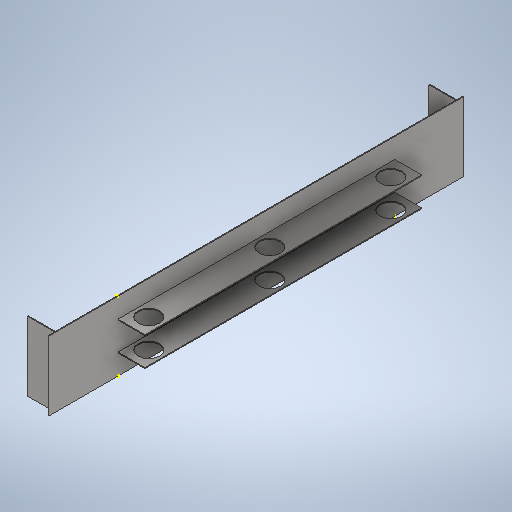
# Autodesk Inventor part: claw platform
Saved by Autodesk Inventor 2025.2 (Build 292293000, 293)
## iProperties
Created: 2025-02-04
Part Number: claw platform
Material: Steel, Galvanized
Document SubType Name: Sheet Metal
Designer: nandu
Density: 7.85 g/cm^3
Sheet Metal Rule: Default_mm
Appearance: Galvanized
Author: nandu
Autodesk Inventor part; units mm, degrees
ref_plane "YZ Plane" through (0, 0, 0) normal (1, 0, 0) x (0, 1, 0)
ref_plane "XZ Plane" through (0, 0, 0) normal (0, 1, 0) x (-1, 0, 0)
ref_plane "XY Plane" through (0, 0, 0) normal (0, 0, 1) x (1, 0, 0)
sketch "Sketch1" plane through (0, 0, 0) normal (1, 0, 0) x (0, 1, 0)
  line L0 (0, 0) -> (50, 0)
  line L1 (50, 0) -> (50, -200)
  line L2 (50, -200) -> (0, -200)
  line L3 (0, -200) -> (0, 0)
  dimension "d0" = 50
  dimension "d1" = 200
  constraints: 8 end point, 2 parallel, 1 horizontal, 1 perpendicular
  measures "d0" distance of L1.end L2.end
  measures "d1" distance of L0.end L1.end
extrude "Extrusion1" add sketch "Sketch1" along normal blind 0.602
sketch "Sketch2" plane through (0.602, 0, 0) normal (1, 0, 0) x (0, 0, -1)
  line L0 (200, 50) -> (0, 50) projected
  line L1 (0, 50) -> (100, 50)
  line L2 (100, 50) -> (100, 35)
  line L3 (0, 0) -> (100, 0)
  line L4 (100, 0) -> (100, 15)
  line L5 (100, 35) -> (200, 35)
  line L6 (200, 0) -> (200, 50) projected
  line L7 (200, 35) -> (200, 35.602)
  line L8 (200, 35.602) -> (0, 35.602)
  line L9 (0, 50) -> (0, 0) projected
  line L10 (0, 35.602) -> (0, 35)
  line L11 (0, 35) -> (100, 35)
  line L12 (100, 15) -> (200, 15)
  line L13 (200, 15) -> (200, 14.398)
  line L14 (200, 14.398) -> (0, 14.398)
  line L15 (0, 14.398) -> (0, 15)
  line L16 (0, 15) -> (100, 15)
  dimension "d4" = 100
  dimension "d5" = 15
  dimension "d6" = 100
  dimension "d7" = 15
  dimension "d9" = 200
  dimension "d13" = 200
  constraints: 28 end point, 6 point on line, 5 perpendicular, 2 horizontal, 1 midpoint, 1 parallel
  measures "d4" distance of L0.end L1.end
  measures "d5" distance of L1.end L2.end
  measures "d6" distance of L3.start L3.end
  measures "d7" distance of L3.end L4.end
  measures "d9" distance of L7.end L8.end
  measures "d13" distance of L13.end L14.end
extrude "Extrusion2" add sketch "Sketch2" along normal blind 19.398 contours L6 L5 L2 L8 | L2 L11 L9 L8 | L6 L14 L4 L12 | L4 L14 L9 L16
sketch "Sketch4" plane through (0.602, 35.602, 0) normal (0, 1, 0) x (1, 0, 0)
  line L0 (-0.602, 0) -> (0, 0) projected
  line L1 (0, 0) -> (0, 12.5)
  line L2 (0, 5) -> (0, 0) projected
  line L3 (0, 12.5) -> (9.699, 12.5)
  line L4 (9.699, 12.5) -> (9.699, 100)
  line L5 (9.699, 100) -> (9.699, 187.5)
  circle A0 centre (9.699, 12.5) radius 7.75
  circle A1 centre (9.699, 100) radius 7.75
  circle A2 centre (9.699, 187.5) radius 7.75
  dimension "d33" = 12.5
  dimension "d34" = 9.699
  dimension "d39" = 15.5
  dimension "d40" = 15.5
  dimension "d41" = 15.5
  dimension "d49" = 87.5
  dimension "d50" = 87.5
  constraints: 8 end point, 3 centre point, 3 coincident, 2 collinear, 2 perpendicular
  measures "d33" distance of L0.end L1.end
  measures "d34" distance of L1.end L3.end
  measures "d39" diameter of A0
  measures "d40" diameter of A1
  measures "d41" diameter of A2
  measures "d49" distance of L5.end L4.end
  measures "d50" distance of L3.end L4.end
extrude "Extrusion4" cut sketch "Sketch4" against normal through all
sketch "Sketch6" plane through (0.602, 15, -200) normal (0, 0, -1) x (-1, 0, 0)
  point P0 (0.602, -15)
sketch "Sketch7" plane through (0, 0, -200) normal (0, 0, -1) x (-1, 0, 0)
  point P0 (0, 0)
sketch "Sketch8" plane through (0, 0, -200) normal (0, 0, -1) x (-1, 0, 0)
  line L0 (-0.602, 50) -> (-0.602, 35.602) projected
  line L1 (-0.602, 50) -> (-0.602, 0)
  line L2 (-0.602, 0) -> (0, 0)
  line L3 (0, 0) -> (0, 50)
  line L4 (0, 50) -> (-0.602, 50)
  constraints: 8 end point, 3 perpendicular, 1 vertical
extrude "Extrusion6" add sketch "Sketch8" along normal blind 50
sketch "Sketch9" plane through (0, 0, 0) normal (0, 0, 1) x (1, 0, 0)
  line L0 (0, 0) -> (0, 50) projected
  line L1 (0, 0) -> (0, 50)
  line L2 (0, 50) -> (0.602, 50)
  line L3 (0.602, 50) -> (0.602, 0)
  line L4 (0.602, 0) -> (0, 0)
  dimension "d53" = 0.602
  constraints: 8 end point, 2 perpendicular, 1 parallel, 1 vertical
  measures "d53" distance of L0.end L2.end
extrude "Extrusion7" add sketch "Sketch9" along normal blind 50
sketch "Sketch10" plane through (0, 0, 0) normal (-1, 0, 0) x (0, 0, 1)
  line L0 (0, 0) -> (-100, 0)
  line L1 (-250, 0) -> (50, 0) projected
  line L2 (-100, 0) -> (-100, 25)
  line L3 (-100, 25) -> (45, 25)
  line L4 (-100, 25) -> (-245, 25)
  line L5 (45.301, 50) -> (44.699, 50)
  line L6 (44.699, 50) -> (44.699, 0)
  line L7 (44.699, 0) -> (45.301, 0)
  line L8 (45.301, 0) -> (45.301, 50)
  line L9 (45.301, 50) -> (44.699, 0) construction
  line L10 (44.699, 50) -> (45.301, 0) construction
  line L11 (-245.301, 50) -> (-244.699, 50)
  line L12 (-244.699, 50) -> (-244.699, 0)
  line L13 (-244.699, 0) -> (-245.301, 0)
  line L14 (-245.301, 0) -> (-245.301, 50)
  line L15 (-245.301, 50) -> (-244.699, 0) construction
  line L16 (-244.699, 50) -> (-245.301, 0) construction
  dimension "d56" = 100
  dimension "d57" = 25
  dimension "d58" = 145
  dimension "d59" = 145
  dimension "d60" = 0.602
  dimension "d61" = 50
  dimension "d62" = 0.602
  dimension "d63" = 50
  constraints: 32 end point, 5 midpoint, 4 parallel, 4 perpendicular, 3 horizontal
  measures "d56" distance of L0.start L0.end
  measures "d57" distance of L0.end L2.end
  measures "d58" distance of L2.end L3.end
  measures "d59" distance of L2.end L4.end
  measures "d60" distance of L7.end L6.end
  measures "d61" distance of L6.end L5.end
  measures "d62" distance of L12.end L13.end
  measures "d63" distance of L11.end L12.end
extrude "Extrusion8" add sketch "Sketch10" along normal blind 19.398 contours L6 L5 L8 L1 | L1 L14 L11 L12
sketch "Sketch11" plane through (0, 0, 45.301) normal (0, 0, 1) x (1, 0, 0)
  line L0 (0, 0) -> (-19.398, 0) projected
  line L1 (-19.398, 50) -> (-19.398, 0) projected
  line L2 (-19.398, 0) -> (-19.398, 10)
  line L3 (-19.398, 10) -> (-9.699, 10)
  line L4 (-9.699, 10) -> (-9.699, 40)
  circle A0 centre (-9.699, 10) radius 7.75
  circle A1 centre (-9.699, 40) radius 7.75
  dimension "d71" = 10
  dimension "d72" = 30
  dimension "d73" = 15.5
  dimension "d74" = 15.5
  constraints: 6 end point, 2 centre point, 2 coincident, 1 horizontal, 1 perpendicular, 1 point on line
  measures "d71" distance of L0.end L2.end
  measures "d72" distance of L3.end L4.end
  measures "d73" diameter of A0
  measures "d74" diameter of A1
extrude "Extrusion9" [suppressed]
sketch "Sketch12" plane through (0.602, 0, 0) normal (1, 0, 0) x (0, 0, -1)
  point P0 (0, 0)
sketch "Sketch13" plane through (0.602, 50, 50) normal (0, 1, 0) x (1, 0, 0)
  point P0 (-0.602, 50)
sketch "Sketch14" plane through (0.602, 50, 50) normal (0, 1, 0) x (1, 0, 0)
  point P0 (-0.602, 50)
sketch "Sketch15" plane through (0, 0, 0) normal (-1, 0, 0) x (0, 0, 1)
  point P0 (0, 0)
equation "\"BendRadius\" = Thickness"
equation "\"BendReliefWidth\" = Thickness"
equation "\"BendReliefDepth\" = 0.5 * Thickness"
equation "\"CornerReliefSize\" = 4 * Thickness"
equation "\"MinimumRemnant\" = 2 * Thickness"
equation "\"TransitionRadius\" = BendRadius"
equation "\"JacobiRadiusSize\" = BendRadius"
equation "\"GapSize\" = Thickness"
equation "\"Thickness\" = 0.602"
body "Solid1"
